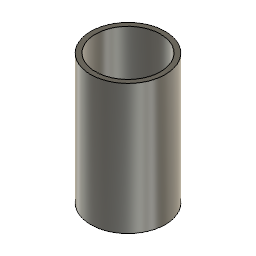
simple-leg (Autodesk Fusion 360 design; units mm, degrees)
Autodesk Fusion 360 part; units mm, degrees
sketch "Skizze1" plane through (0, 0, 0) normal (0, 0, 1) x (1, 0, 0)
  circle A0 centre (0, 0) radius 23
  circle A1 centre (0, 0) radius 20.025
extrude "Extrusion1" add sketch "Skizze1" against normal blind 80
equation "leg_outer_diameter = 46 mm" comment "Aussendurchmesser der Röhre"
equation "leg_inner_diameter = 40.05 mm" comment "Innendurchmesser der Röhre"
equation "leg_length = 80 mm" comment "Laenge der Röhre"
equation "d4 = -leg_length"
named bodies: "Parametric_Tetrapod_Leg_Pipe"
